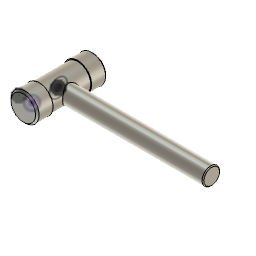
tpu_mallet (Autodesk Fusion 360 design; units mm, degrees)
part number: 2025-08-12-14-59-03-483
Autodesk Fusion 360 part; units mm, degrees
sketch "Sketch1" plane through (0, 0, 0) normal (0, 1, 0) x (1, 0, 0)
  circle A0 centre (0, 0) radius 15
  dimension "d5" = 30
  constraint coincident A0.centre origin
  measures "d5" diameter of A0
extrude "Extrude1" add sketch "Sketch1" along normal mid plane 60 makes body 1
sketch "Sketch2" plane through (0, -30, 0) normal (0, -1, 0) x (1, 0, 0)
  circle A0 centre (0, 0) radius 15
  line L0 (0, 0) -> (-15, 0) construction
  constraint coincident A0.centre L0.start
  constraint coincident A0 L0.end
  constraint horizontal L0
ref_plane "WorkPlane1" through (0, -30, 0) normal (-1, 0, 0) x (0, -1, 0)
sketch "Sketch3" plane through (0, -30, 0) normal (-1, 0, 0) x (0, -1, 0)
  line L0 (0, 0) -> (0, 12)
  line L1 (0, 12) -> (-5, 12)
  line L2 (-5, 12) -> (-5, 11)
  line L3 (-5, 11) -> (-8, 11)
  line L4 (-8, 11) -> (-8, 16)
  line L5 (-8, 16) -> (10, 16)
  line L6 (10, 16) -> (10, 0)
  line L7 (10, 0) -> (0, 0)
  line L8 (-5, 12) -> (-6, 11)
  line L9 (-7, 11) -> (-8, 12)
  dimension "d11" = 12
  dimension "d13" = 5
  dimension "d14" = 1
  dimension "d15" = 3
  dimension "d16" = 5
  dimension "d17" = 18
  dimension "d18" = 45
  dimension "d19" = 45
  dimension "d20" = 1
  constraint coincident L0.start L7.end
  constraint vertical L0
  constraint perpendicular L0 L1
  constraint perpendicular L1 L2
  constraint perpendicular L2 L3
  constraint perpendicular L3 L4
  constraint perpendicular L4 L5
  constraint perpendicular L5 L6
  constraint perpendicular L0 L7
  constraint coincident L3 L8.end
  constraint coincident L3 L9.start
  constraint coincident L4 L9.end
  measures "d11" distance of L0.start L0.end
  measures "d13" distance of L0.end L1.end
  measures "d14" distance of L1.end L2.end
  measures "d15" distance of L2.end L3.end
  measures "d16" distance of L3.end L4.end
  measures "d17" distance of L4.end L5.end
  measures "d18" angle of L2 L8
  measures "d19" angle of L4 L9
  measures "d20" distance of L3.end L9.end
revolve "Revolve1" add sketch "Sketch3" angle 360 about axis through (0, -40, 0) along (0, 1, 0) separate body contours L0 L1 L3 L4 L5 L6 L7 L8 L9 makes body 2
chamfer "Chamfer1" distance 2 angle 45 1 edges at (-14.9172, -40, -5.7858) on bodies 2
sketch "Sketch4" plane through (0, 0, 0) normal (1, 0, 0) x (0, 1, 0)
  circle A0 centre (0, 0) radius 2.5
  circle A1 centre (0, 0) radius 10
  dimension "d26" = 5
  dimension "d33" = 20
  constraint coincident A0.centre A1.centre
  measures "d26" diameter of A0
  measures "d33" diameter of A1
sketch "Sketch5" plane through (0, 0, 0) normal (1, 0, 0) x (0, 1, 0)
extrude "Extrude2" cut sketch "Sketch4" along normal blind 15 and the other way blind 7.5 contours A0 bodies 1
mirror "Mirror1" about plane through (0, 0, 0) normal (0, 1, 0) of bodies 2 makes body 3
combine "Combine1" operation cut target body 1 tool bodies 2 3 keep tools
extrude "Extrude3" cut sketch "Sketch4" along normal blind 10 from surface at 10 bodies 1
thread "Thread1" "ISO Metric Trapezoidal Threads 18.0 TR18x4 TR18x4 7H" major diameter 18.5 minor diameter 14.1875 pitch 4 angle 30 modelled right hand crest width 1.4668 on face at (4.1667, 2.4876, -0.2489) crest through (-6.5, 7.0938, 0) on bodies 1
extrude "Extrude4" add sketch "Sketch4" along normal blind 175 and the other way blind 7.5 separate body contours A0 | A1 makes body 4
extrude "Extrude5" cut sketch "Sketch4" along normal up to surface (10 mm away) and the other way blind 10 bodies 4
thread "Thread2" "ISO Metric Trapezoidal Threads 18.0 TR18x4 TR18x4 7e" major diameter 17.85 minor diameter 13.287 pitch 4 angle 30 modelled right hand crest width 1.4433 on face at (4.1667, 2.4876, -0.2489) crest through (-8.5, 8.925, 0) on bodies 4
chamfer "Chamfer2" distance 1 angle 45 1 edges at (175, -9.3233, -3.6162) on bodies 4
equation "hammer_diameter = 30 mm"
equation "hammer_hard_length = 60 mm" comment "includes attachment portion"
equation "TPU_length = 10 mm" comment "does not include attachment"
equation "attachment_length = 8 mm"
equation "d5 = hammer_diameter"
equation "d6 = hammer_hard_length"
equation "tpu_hook_depth = 1 mm"
equation "tpu_grip_width = 3 mm"
equation "d11 = hammer_diameter / 2 - tpu_grip_width"
equation "tpu_hook_length = 4 mm"
equation "d13 = attachment_length - tpu_grip_width"
equation "d14 = tpu_hook_depth"
equation "d15 = tpu_grip_width"
equation "d16 = tpu_hook_depth + tpu_grip_width + tpu_extra_width"
equation "d17 = attachment_length + TPU_length"
equation "d20 = tpu_hook_depth"
equation "tpu_extra_width = 1 mm"
equation "handle_insertion_diameter = 17 mm"
equation "handle_diameter = 20 mm"
equation "d27 = hammer_diameter / 2"
equation "d29 = hammer_diameter / 4"
equation "d33 = handle_diameter"
equation "d34 = hammer_diameter / 3"
equation "d35 = hammer_diameter / 3"
equation "d45 = hammer_diameter / 4"
named bodies: "head", "handle"
